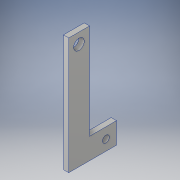
# Autodesk Inventor part: PaddleCollection2.1AxleSupport
Saved by Autodesk Inventor 2019 (Build 230136000, 136)
## iProperties
Created: 2018-10-20
Part Number: PaddleCollection2.1AxleSupport
Material: Aluminum 6061
Document SubType Name: Modeling
Designer: User
Density: 2.7 g/cm^3
Appearance: Aluminum - Flat
Author: User
Autodesk Inventor part; units mm, degrees
ref_plane "YZ Plane" through (0, 0, 0) normal (1, 0, 0) x (0, 1, 0)
ref_plane "XZ Plane" through (0, 0, 0) normal (0, 1, 0) x (-1, 0, 0)
ref_plane "XY Plane" through (0, 0, 0) normal (0, 0, 1) x (1, 0, 0)
sketch "Sketch1" plane through (0, 0, 0) normal (1, 0, 0) x (0, 1, 0)
  line L0 (0, 0) -> (139.7, 0)
  line L1 (139.7, 0) -> (139.7, -57.15)
  line L2 (139.7, -57.15) -> (0, -57.15)
  line L3 (0, -57.15) -> (0, 0)
  circle A0 centre (127, -12.1412) radius 6.35
  circle A1 centre (12.7, -44.45) radius 4.064
  line L4 (139.7, -57.15) -> (25.4, -57.15)
  line L5 (25.4, -57.15) -> (25.4, -24.8412)
  line L6 (25.4, -24.8412) -> (139.7, -24.8412)
  line L7 (139.7, -24.8412) -> (139.7, -57.15)
  dimension "d0" = 139.7
  dimension "d1" = 57.15
  dimension "d2" = 12.7
  dimension "d3" = 8.128
  dimension "d4" = 32.3088
  dimension "d5" = 114.3
  dimension "d6" = 12.7
  dimension "d7" = 12.7
  dimension "d8" = 12.7
  dimension "d9" = 12.7
  constraints: 16 end point, 4 parallel, 2 centre point, 2 horizontal, 2 perpendicular
  measures "d0" distance of L1.end L2.end
  measures "d1" distance of L0.end L1.end
  measures "d2" diameter of A0
  measures "d3" diameter of A1
  measures "d4" vertical distance of A1.centre A0.centre
  measures "d5" horizontal distance of A1.centre A0.centre
  measures "d6" distance from line of L2 A1.centre
  measures "d7" distance from line of L3 A1.centre
  measures "d8" distance from line of A0.centre L6
  measures "d9" distance from line of A1.centre L5
extrude "Extrusion1" add sketch "Sketch1" along normal blind 6.35 contours L0 L1 L6 L5 L2 L3
body "Solid1"
